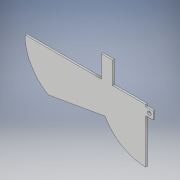
# Autodesk Inventor part: CollectionCasing
Saved by Autodesk Inventor 2019 (Build 230136000, 136)
## iProperties
Created: 2018-10-04
Part Number: CollectionCasing
Material: Generic
Document SubType Name: Modeling
Designer: User
Density: 1 g/cm^3
Appearance: Default
Author: User
Autodesk Inventor part; units mm, degrees
ref_plane "YZ Plane" through (0, 0, 0) normal (1, 0, 0) x (0, 1, 0)
ref_plane "XZ Plane" through (0, 0, 0) normal (0, 1, 0) x (-1, 0, 0)
ref_plane "XY Plane" through (0, 0, 0) normal (0, 0, 1) x (1, 0, 0)
sketch "Sketch1" plane through (0, 0, 0) normal (0, 0, 1) x (1, 0, 0)
  arc A0 (0, 0) -> (39.7002, -68.7324) centre (79.375, 0.0157) ccw
  line L0 (39.7002, -68.7324) -> (139.7567, -51.0897)
  line L1 (39.7002, -68.7324) -> (141.3002, -68.7324) construction
  arc A1 (136.4379, -51.6749) -> (205.7416, -92.3565) centre (205.743, -12.9815) ccw
  arc A2 (139.7567, -51.0897) -> (205.7416, -89.1815) centre (205.743, -12.9815) ccw
  line L2 (205.7416, -89.1815) -> (205.7416, -92.3565)
  line L3 (0, 0) -> (205.7416, 0)
  line L4 (205.7416, 0) -> (205.7416, -89.1815)
  dimension "d0" = 79.375
  dimension "d1" = 68.7324
  dimension "d2" = 39.7002
  dimension "d3" = 101.6
  dimension "d4" = 10
  dimension "d5" = 79.375
  dimension "d6" = 76.2
  dimension "d7" = 3.175
  dimension "d9" = 0
  dimension "d10" = 0
  dimension "d11" = 48.9712
  constraints: 10 end point, 6 point on circle, 3 centre point, 2 horizontal, 1 concentric, 1 equal length, 1 perpendicular, 1 point on line, 1 vertical
  measures "d0" radius of A0
  measures "d1" vertical distance of L3.start L0.start
  measures "d2" horizontal distance of L3.start L0.start
  measures "d3" distance of L0.start L0.end
  measures "d4" angle of L1 L0
  measures "d5" radius of A1
  measures "d6" radius of A2
  measures "d7" distance of L2.end L2.start
  measures "d9" distance of L0.end A2.start
  measures "d10" distance of L0.end A2.start
  measures "d11" distance from line of L2.start L0
extrude "Extrusion1" add sketch "Sketch1" along normal blind 3.175
sketch "Sketch2" plane through (0, 0, 3.175) normal (0, 0, 1) x (1, 0, 0)
  line L0 (205.7416, -92.3565) -> (205.7416, 0) projected
  line L1 (205.7416, -3.4565) -> (218.4416, -3.4565)
  line L2 (218.4416, -3.4565) -> (218.4416, -16.1565)
  line L3 (218.4416, -16.1565) -> (205.7416, -16.1565)
  line L4 (205.7416, -16.1565) -> (205.7416, -3.4565)
  circle A0 centre (212.0916, -9.8065) radius 3.175
  point P0 (0, 0)
  dimension "d14" = 12.7
  dimension "d15" = 12.7
  dimension "d16" = 92.3565
  dimension "d17" = 6.35
  dimension "d18" = 82.55
  dimension "d19" = 6.35
  constraints: 8 end point, 2 parallel, 1 centre point, 1 horizontal, 1 perpendicular, 1 point on line
  measures "d14" distance of L2.end L3.end
  measures "d15" distance of L1.end L2.end
  measures "d16" distance of L0.start L0.end
  measures "d17" diameter of A0
  measures "d18" vertical distance of L0.start A0.centre
  measures "d19" distance from line of A0.centre L3
extrude "Extrusion2" add sketch "Sketch2" against normal blind 3.175
sketch "Sketch3" plane through (0, 0, 3.175) normal (0, 0, 1) x (1, 0, 0)
  circle A0 centre (212.0916, -9.8065) radius 3.175 projected
  arc A1 (0, 0) -> (39.7002, -68.7324) centre (79.375, 0.0157) ccw projected
  line L0 (39.7002, -68.7324) -> (136.4379, -51.6749) projected
  arc A2 (136.4379, -51.6749) -> (205.7416, -92.3565) centre (205.743, -12.9815) ccw projected
  line L1 (205.7416, -92.3565) -> (205.7416, -16.1565) projected
  line L2 (218.4416, -16.1565) -> (205.7416, -16.1565) projected
  line L3 (218.4416, -3.4565) -> (218.4416, -16.1565) projected
  line L4 (205.7416, -3.4565) -> (218.4416, -3.4565) projected
  line L5 (205.7416, -3.4565) -> (205.7416, 0) projected
  line L6 (205.7416, 0) -> (0, 0) projected
  line L7 (205.7416, 0) -> (0, 0) projected
  line L8 (149.3513, 0) -> (130.3013, 0)
  line L9 (130.3013, 0) -> (130.3013, 37.2251)
  line L10 (130.3013, 37.2251) -> (149.3513, 37.2251)
  line L11 (149.3513, 37.2251) -> (149.3513, 0)
  dimension "d22" = 19.05
  dimension "d23" = 88.9
  dimension "d25" = 47.0315
  dimension "d26" = 62.7403
  constraints: 8 end point, 2 parallel, 1 horizontal, 1 perpendicular, 1 point on line
  measures "d22" distance of L9.end L10.end
  measures "d23" distance from line of L10 L0.end
  measures "d25" distance from line of A0.centre L10
  measures "d26" horizontal distance of A0.centre L10.end
extrude "Extrusion3" add sketch "Sketch3" against normal blind 3.175 contours L9 L10 L11 L6
equation "\"d19\" = 0.5 * d15"
body "Solid1"
